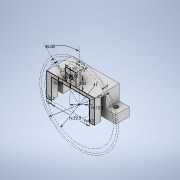
# Autodesk Inventor part: FS90-Mount1
Saved by Autodesk Inventor 2022 (Build 260153000, 153)
## iProperties
Created: 2024-06-14
Part Number: FS90-Mount1
Material: 一般
Document SubType Name: Modeling
Designer: yamashita1
Density: 1 g/cm^3
Appearance: 既定
Author: yamashita1
Autodesk Inventor part; units mm, degrees
ref_plane "YZ Plane" through (0, 0, 0) normal (1, 0, 0) x (0, 1, 0)
ref_plane "XZ Plane" through (0, 0, 0) normal (0, 1, 0) x (-1, 0, 0)
ref_plane "XY Plane" through (0, 0, 0) normal (0, 0, 1) x (1, 0, 0)
derived "FS90R.ipt"
sketch "スケッチ2" plane through (0, 0, 0) normal (0, 0, 1) x (1, 0, 0)
  circle A0 centre (0, 0) radius 6.05 construction
  line L0 (-16.45, 6.05) -> (6.05, 6.05) construction
  line L1 (6.05, 6.05) -> (6.05, -6.05) construction
  line L2 (6.05, -6.05) -> (-16.45, -6.05) construction
  line L3 (-16.45, -6.05) -> (-16.45, 6.05) construction
  line L4 (-16.65, -6.05) -> (-19.45, -6.05)
  line L5 (-19.45, -6.05) -> (-19.45, 8.05)
  line L6 (-19.45, 8.05) -> (9.05, 8.05)
  line L7 (9.05, 8.05) -> (9.05, -6.05)
  line L8 (9.05, -6.05) -> (6.25, -6.05)
  line L9 (6.25, -6.05) -> (6.25, 6.25)
  line L10 (6.25, 6.25) -> (-16.65, 6.25)
  line L11 (-16.65, 6.25) -> (-16.65, -6.05)
  circle A1 centre (0, 0) radius 23.5 construction
  line L12 (0, 0) -> (0, 30.3391) construction
  line L13 (-21.7931, 21.7931) -> (0, 0) construction
  circle A2 centre (0, 0) radius 20.5 construction
  line L14 (-4.843, 20.5) -> (4.843, 20.5) construction
  line L15 (-1.35, 22.2) -> (1.35, 22.2) construction
  line L16 (1.35, 22.2) -> (1.35, 18.8) construction
  line L17 (1.35, 18.8) -> (-1.35, 18.8) construction
  line L18 (-1.35, 18.8) -> (-1.35, 22.2) construction
  line L19 (-17.1178, 11.8736) -> (-11.8736, 17.1178) construction
  line L20 (-16.6524, 14.7432) -> (-14.7432, 16.6524) construction
  line L21 (-14.7432, 16.6524) -> (-12.339, 14.2482) construction
  line L22 (-12.339, 14.2482) -> (-14.2482, 12.339) construction
  line L23 (-14.2482, 12.339) -> (-16.6524, 14.7432) construction
  circle A3 centre (0, 0) radius 22.5 construction
  circle A4 centre (-5.08, 11.86) radius 1.1
  circle A5 centre (-5.08, 11.86) radius 2.5 construction
  line L24 (-8.255, 8.05) -> (-1.905, 8.05)
  line L25 (-1.905, 8.05) -> (-1.905, 15.67)
  line L26 (-1.905, 15.67) -> (-8.255, 15.67)
  line L27 (-8.255, 15.67) -> (-8.255, 8.05)
  line L28 (-5.08, 17.5367) -> (-5.08, 4.1408) construction
  point P0 (0, 20.5)
  point P1 (0, 22.2)
  point P2 (-1.35, 20.5)
  point P3 (-14.4957, 14.4957)
  point P4 (-15.6978, 15.6978)
  point P5 (-13.5411, 15.4503)
  point P6 (-5.08, 15.67)
  dimension "d18" = 12.1
  dimension "d19" = 22.5
  dimension "CLEARANCE" = 0.2
  dimension "d21" = 0.2
  dimension "d22" = 0.2
  dimension "d24" = 3
  dimension "d25" = 2
  dimension "d39" = 47
  dimension "d40" = 45
  dimension "d41" = 2.7
  dimension "d42" = 3.4
  dimension "d43" = 41
  dimension "d44" = 1
  dimension "d46" = 2.2
  dimension "d47" = 5.08
  dimension "d48" = 3.81
  dimension "d49" = 5
  dimension "d50" = 6.35
  dimension "d51" = 7.62
  constraints: 58 end point, 12 perpendicular, 11 point on line, 9 parallel, 7 midpoint, 6 centre point, 5 coincident, 5 horizontal, 5 tangent, 3 equal length, 1 collinear, 1 vertical
  measures "d18" diameter of A0
  measures "d19" distance of L1.end L2.end
  measures "CLEARANCE" distance between parallel lines of L3 L11
  measures "d21" distance between parallel lines of L10 L0
  measures "d22" distance between parallel lines of L1 L9
  measures "d24" distance between parallel lines of L3 L5
  measures "d25" distance between parallel lines of L0 L6
  measures "d39" diameter of A1
  measures "d40" angle of L13 L12
  measures "d41" distance of L16.end L17.end
  measures "d42" distance of L15.end L16.end
  measures "d43" diameter of A2
  measures "d44" radial gap between concentric circles of A1 A3
  measures "d46" diameter of A4
  measures "d47" distance from line of L12 A4.centre
  measures "d48" distance from line of L6 A4.centre
  measures "d49" diameter of A5
  measures "d50" distance of L25.end L26.end
  measures "d51" distance of L24.end L25.end
extrude "ベース" add sketch "スケッチ2" against normal blind 15 contours L4 L5 L6 L7 L8 L9 L10 L11
sketch "スケッチ3" plane through (9.05, -6.05, 0) normal (1, 0, 0) x (0, 0, -1)
  line L0 (5.45, 18.1341) -> (5.45, -3.0415) construction
  line L1 (0, 0) -> (0, 14.1) construction
  line L2 (4, 0) -> (6.9, 0)
  line L3 (6.9, 0) -> (6.9, 12.3)
  line L4 (6.9, 12.3) -> (4, 12.3)
  line L5 (4, 12.3) -> (4, 0)
  line L6 (0, 12.3) -> (15, 12.3) projected
  line L7 (0, 0) -> (15, 0) projected
  point P0 (0, 6.05)
  point P1 (5.45, 12.3)
  dimension "d28" = 5.45
  dimension "d29" = 2.9
  constraints: 10 end point, 2 collinear, 2 parallel, 1 horizontal, 1 midpoint, 1 perpendicular, 1 point on line, 1 vertical
  measures "d28" distance between parallel lines of L0 L1
  measures "d29" distance of L3.end L4.end
extrude "タブ切欠き" cut sketch "スケッチ3" against normal through all
sketch "スケッチ4" plane through (6.25, -6.05, -15) normal (0, -1, 0) x (1, 0, 0)
  line L0 (0, 8.1) -> (0, 0) projected
  line L1 (0, 0) -> (8.8, 0)
  line L2 (8.8, 0) -> (8.8, 8.1)
  line L3 (8.8, 8.1) -> (0, 8.1)
  line L4 (0, 8.1) -> (0, 0)
  line L5 (-22.9, 0) -> (-31.7, 0)
  line L6 (-31.7, 0) -> (-31.7, 8.1)
  line L7 (-31.7, 8.1) -> (-22.9, 8.1)
  line L8 (-22.9, 8.1) -> (-22.9, 0)
  line L9 (-22.9, 8.1) -> (-22.9, 0) projected
  line L10 (2.8, 8.1) -> (0, 8.1) projected
  line L11 (4.8, 18.5805) -> (4.8, -5.7068) construction
  line L12 (-27.7, -5.7068) -> (-27.7, 14.4988) construction
  line L13 (-33.2224, 4) -> (10.563, 4) construction
  circle A0 centre (4.8, 4) radius 1.35
  circle A1 centre (-27.7, 4) radius 1.35
  point P0 (-6.25, 15)
  dimension "d32" = 8.8
  dimension "d33" = 11.05
  dimension "d34" = 21.45
  dimension "d35" = 11
  dimension "d36" = 2.7
  constraints: 22 end point, 6 point on line, 4 parallel, 3 collinear, 3 horizontal, 2 centre point, 2 perpendicular, 2 vertical, 1 equal radius
  measures "d32" distance of L0.end L1.end
  measures "d33" distance from line of L11 point (-6.25, 15)
  measures "d34" distance from line of L12 point (-6.25, 15)
  measures "d35" vertical distance of L13.end point (-6.25, 15)
  measures "d36" diameter of A0
extrude "マウント" add sketch "スケッチ4" against normal blind 5
extrude "押し出し5" add sketch "スケッチ2" against normal blind 3 contours L27 L26 L25 L6
equation "\"d18\" = HEIGHT"
equation "\"d19\" = WIDTH"
equation "\"d21\" = CLEARANCE"
equation "\"d22\" = CLEARANCE"
equation "\"d29\" = TAB_THIN + 2 * CLEARANCE"
equation "\"d32\" = MOUNT_WIDTH - CLEARANCE"
equation "\"MOUNT_WIDTH\" = 9"
equation "\"HEIGHT\" = 12.1"
equation "\"WIDTH\" = 22.5"
equation "\"TAB_THIN\" = 2.5"
